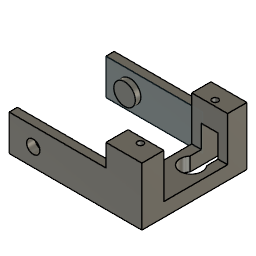
leg connector sprint 5 (Autodesk Fusion 360 design; units mm, degrees)
Autodesk Fusion 360 part; units mm, degrees
sketch "Sketch1" plane through (0, 0, 0) normal (0, 0, 1) x (1, 0, 0)
  line L0 (6.5, -11.5) -> (-6.5, -11.5)
  line L1 (-6.5, -11.5) -> (-6.5, 11.5)
  line L2 (-6.5, 11.5) -> (6.5, 11.5)
  line L3 (6.5, 11.5) -> (6.5, -11.5)
  line L4 (6.5, -11.5) -> (-6.5, 11.5) construction
  line L5 (-6.5, -11.5) -> (6.5, 11.5) construction
  line L6 (6.5, -11.5) -> (-6.5, -11.5)
  line L7 (-6.5, -11.5) -> (-6.5, -17.5)
  line L8 (-6.5, -17.5) -> (6.5, -17.5)
  line L9 (6.5, -17.5) -> (6.5, -11.5)
  line L10 (6.5, 11.5) -> (-6.5, 11.5)
  line L11 (-6.5, 11.5) -> (-6.5, 17.5)
  line L12 (-6.5, 17.5) -> (6.5, 17.5)
  line L13 (6.5, 17.5) -> (6.5, 11.5)
  dimension "d1" = 13
  dimension "d2" = 23
  dimension "d3" = 6
  dimension "d4" = 6
  constraint horizontal L0
  constraint perpendicular L0 L1
  constraint parallel L0 L2
  constraint parallel L1 L3
  constraint coincident L4 origin
  constraint coincident L5 origin
  constraint horizontal L6
  constraint vertical L7
  constraint horizontal L8
  constraint vertical L9
  constraint horizontal L10
  constraint vertical L11
  constraint horizontal L12
  constraint vertical L13
  measures "d1" distance of L1.end L2.end
  measures "d2" distance of L0.end L1.end
  measures "d3" distance of L0.start L8.end
  measures "d4" distance of L2.end L12.end
extrude "Extrude1" add sketch "Sketch1" along normal blind 21 contours L0 L6 L7 L8 L9 | L2 L10 L11 L12 L13 makes body 1 at (-2.1667, -17.5, 7) makes body 2 at (-2.1667, 17.5, 7)
extrude "Extrude2" add sketch "Sketch1" along normal blind 5 contours L0 L1 L2 L3 L6 L10 bodies 1 2
sketch "Sketch2" plane through (0, 0, 5) normal (0, 0, 1) x (-1, 0, 0)
  line L0 (-6.5, 11.5) -> (-6.5, -11.5)
  line L1 (-6.5, -11.5) -> (6.5, -11.5)
  line L2 (6.5, -11.5) -> (6.5, 11.5)
  line L3 (6.5, 11.5) -> (-6.5, 11.5)
  circle A0 centre (0, -5.75) radius 4
  dimension "d9" = 8
  measures "d9" diameter of A0
extrude "Extrude3" cut sketch "Sketch2" against normal blind 6.5 contours A0 bodies 1
sketch "Sketch3" plane through (-6.5, 0, 0) normal (-1, 0, 0) x (0, -1, 0)
  line L0 (-17.5, 0) -> (17.5, 0)
  line L1 (17.5, 0) -> (17.5, 21)
  line L2 (17.5, 21) -> (11.5, 21)
  line L3 (11.5, 21) -> (11.5, 5)
  line L4 (11.5, 5) -> (-11.5, 5)
  line L5 (-11.5, 5) -> (-11.5, 21)
  line L6 (-11.5, 21) -> (-17.5, 21)
  line L7 (-17.5, 21) -> (-17.5, 0)
  line L8 (-17.5, 0) -> (-14.5, 0)
  line L9 (-14.5, 0) -> (-14.5, 13)
  line L10 (-14.5, 13) -> (-17.5, 13)
  line L11 (-17.5, 13) -> (-17.5, 0)
  line L12 (17.5, 0) -> (14.5, 0)
  line L13 (14.5, 0) -> (14.5, 13)
  line L14 (14.5, 13) -> (17.5, 13)
  line L15 (17.5, 13) -> (17.5, 0)
  dimension "d12" = 3
  constraint horizontal L8
  constraint vertical L9
  constraint horizontal L10
  constraint vertical L11
  constraint coincident L0.start L7.end
  constraint horizontal L12
  constraint vertical L13
  constraint horizontal L14
  constraint vertical L15
  constraint coincident L0.end L1.start
  measures "d12" distance of L0.end L12.end
extrude "Extrude4" add sketch "Sketch3" along normal blind 25 contours L0 L7 L8 L9 L10 L11 | L0 L1 L12 L13 L14 L15 bodies 1
chamfer "Chamfer1" distance 2 angle 45 2 edges at (-6.5, 17.5, 17) (-6.5, -17.5, 17) on bodies 1
sketch "Sketch4" plane through (0, -14.5, 0) normal (0, 1, 0) x (-1, 0, 0)
  line L0 (6.5, 13) -> (6.5, 0)
  line L1 (6.5, 0) -> (31.5, 0)
  line L2 (31.5, 0) -> (31.5, 13)
  line L3 (31.5, 13) -> (6.5, 13)
  circle A0 centre (25.25, 6.5) radius 4
  dimension "d16" = 8
  measures "d16" diameter of A0
extrude "Extrude5" add sketch "Sketch4" along normal blind 2 contours A0 bodies 1
sketch "Sketch5" plane through (0, 17.5, 0) normal (0, 1, 0) x (-1, 0, 0)
  line L0 (4.5, 13) -> (4.5, 21)
  line L1 (4.5, 21) -> (-6.5, 21)
  line L2 (-6.5, 21) -> (-6.5, 0)
  line L3 (-6.5, 0) -> (31.5, 0)
  line L4 (31.5, 0) -> (31.5, 13)
  line L5 (31.5, 13) -> (4.5, 13)
  line L6 (-3, -10) -> (3, -10)
  line L7 (3, -10) -> (3, 10)
  line L8 (3, 10) -> (-3, 10)
  line L9 (-3, 10) -> (-3, -10)
  line L10 (-3, -10) -> (3, 10) construction
  line L11 (3, -10) -> (-3, 10) construction
  constraint horizontal L6
  constraint perpendicular L6 L7
  constraint parallel L6 L8
  constraint parallel L7 L9
  constraint coincident L10 origin
  constraint coincident L11 origin
extrude "Extrude6" cut sketch "Sketch5" against normal blind 6 contours L3 L7 L8 L9 bodies 1
extrude "Extrude7" add 2 faces at (-31.5, 16.5, 8.6667) (-31.5, -15.5, 8.6667) along direction (-1, 0, 0) blind 10 on bodies 1 bodies 1
extrude "Extrude8" cut 1 faces at (-26.4956, -12.5, 5.7272) along direction (0, -1, 0) blind 2 on bodies 1 bodies 1
extrude "Extrude9" add 1 faces at (-13.1667, -17.5, 4.3333) along direction (0, -1, 0) blind 5 on bodies 1 bodies 1
extrude "Extrude10" cut 1 faces at (-18.1667, -14.5, 4.3333) along direction (0, -1, 0) blind 2 on bodies 1 bodies 1
extrude "Extrude11" cut 1 faces at (-13.1667, -22.5, 4.3333) along direction (0, 1, 0) blind 3 on bodies 1 bodies 1
sketch "Sketch6" plane through (0, -16.5, 0) normal (0, 1, 0) x (-1, 0, 0)
  line L0 (6.5, 13) -> (6.5, 0)
  line L1 (6.5, 0) -> (41.5, 0)
  line L2 (41.5, 0) -> (41.5, 13)
  line L3 (41.5, 13) -> (6.5, 13)
  line L4 (24, 13) -> (24, 0)
  circle A0 centre (32.75, 6.5) radius 4
  dimension "d31" = 8
  constraint midpoint L3 L4.start
  constraint midpoint L1 L4.end
  measures "d31" diameter of A0
extrude "Extrude12" add sketch "Sketch6" along normal blind 2 contours A0 bodies 1
sketch "Sketch7" plane through (0, 0, 13) normal (0, 0, 1) x (-1, 0, 0)
  line L0 (41.5, 19.5) -> (4.5, 19.5)
  line L1 (4.5, 19.5) -> (4.5, 17.5)
  line L2 (4.5, 17.5) -> (6.5, 15.5)
  line L3 (6.5, 15.5) -> (6.5, 16.5)
  line L4 (6.5, 16.5) -> (41.5, 16.5)
  line L5 (41.5, 16.5) -> (41.5, 19.5)
  line L6 (6.5, 19.5) -> (6.5, 15.5)
  line L7 (6.5, 19.5) -> (4.5, 19.5)
  constraint coincident L0 L6.start
  constraint coincident L2.end L3.start
  constraint coincident L0.end L1.start
extrude "Extrude13" add 1 faces at (-4.5, -18.1667, 15.6667) along direction (-1, 0, 0) blind 2 on bodies 1 bodies 1
extrude "Extrude14" add 1 faces at (-5.8333, -17.5, 15.6667) along direction (0, 1, 0) blind 2 on bodies 1 bodies 1
chamfer "Chamfer2" distance 2 angle 45 1 edges at (-6.5, -19.5, 17) on bodies 1
extrude "Extrude15" cut 1 faces at (-18.1667, 14.5, 4.3333) along direction (0, 1, 0) blind 1 on bodies 1 bodies 1
extrude "Extrude16" add 1 faces at (-16.3333, 17.5, 4.3333) along direction (0, 1, 0) blind 1 on bodies 1 bodies 1
sketch "Sketch8" plane through (0, 15.5, 0) normal (0, -1, 0) x (1, 0, 0)
  line L0 (-6.5, 0) -> (-6.5, 13)
  line L1 (-6.5, 13) -> (-41.5, 13)
  line L2 (-41.5, 13) -> (-41.5, 0)
  line L3 (-41.5, 0) -> (-6.5, 0)
extrude "Extrude17" cut 1 faces at (-31.963, -14.5, 4.8658) along direction (0, 1, 0) blind 38 on bodies 1 bodies 1
sketch "Sketch9" plane through (0, 18.5, 0) normal (0, 1, 0) x (-1, 0, 0)
  circle A0 centre (32.75, 6.5) radius 4
  line L0 (-3, 0) -> (-3, 10)
  line L1 (-3, 10) -> (3, 10)
  line L2 (3, 10) -> (3, 0)
  line L3 (3, 0) -> (41.5, 0)
  line L4 (41.5, 0) -> (41.5, 13)
  line L5 (41.5, 13) -> (4.5, 13)
  line L6 (4.5, 13) -> (4.5, 21)
  line L7 (4.5, 21) -> (-6.5, 21)
  line L8 (-6.5, 21) -> (-6.5, 0)
  line L9 (-6.5, 0) -> (-3, 0)
  circle A1 centre (32.75, 6.5) radius 1.25
  dimension "d45" = 2.5
  constraint concentric A0 A1
  measures "d45" diameter of A1
extrude "Extrude18" add sketch "Sketch9" against normal blind 3 contours A0 bodies 1
extrude "Extrude19" cut 1 faces at (-1, 16.1667, 10) along direction (0, 0, 1) blind 1 on bodies 1 bodies 1
sketch "Sketch10" plane through (0, 0, 21) normal (0, 0, 1) x (-1, 0, 0)
  line L0 (4.5, -17.5) -> (6.5, -15.5)
  line L1 (6.5, -15.5) -> (6.5, -11.5)
  line L2 (6.5, -11.5) -> (-6.5, -11.5)
  line L3 (-6.5, -11.5) -> (-6.5, -18.5)
  line L4 (-6.5, -18.5) -> (4.5, -18.5)
  line L5 (4.5, -18.5) -> (4.5, -17.5)
  circle A0 centre (0, -13.5) radius 1.1
  dimension "d51" = 2.2
  measures "d51" diameter of A0
extrude "Extrude20" cut sketch "Sketch10" against normal blind 4 contours A0 bodies 1
sketch "Sketch11" plane through (0, 0, 21) normal (0, 0, 1) x (-1, 0, 0)
  line L0 (6.5, 17.5) -> (4.5, 19.5)
  line L1 (4.5, 19.5) -> (-6.5, 19.5)
  line L2 (-6.5, 19.5) -> (-6.5, 11.5)
  line L3 (-6.5, 11.5) -> (6.5, 11.5)
  line L4 (6.5, 11.5) -> (6.5, 17.5)
  circle A0 centre (0, 13.5) radius 1.1
  dimension "d55" = 2.2
  measures "d55" diameter of A0
extrude "Extrude21" cut sketch "Sketch11" against normal blind 4 contours A0 bodies 1
sketch "Sketch12" plane through (0, 18.5, 0) normal (0, 1, 0) x (-1, 0, 0)
  line L0 (-3, 0) -> (-3, 11)
  line L1 (-3, 11) -> (3, 11)
  line L2 (3, 11) -> (3, 0)
  line L3 (3, 0) -> (41.5, 0)
  line L4 (41.5, 0) -> (41.5, 13)
  line L5 (41.5, 13) -> (4.5, 13)
  line L6 (4.5, 13) -> (4.5, 21)
  line L7 (4.5, 21) -> (-6.5, 21)
  line L8 (-6.5, 21) -> (-6.5, 0)
  line L9 (-6.5, 0) -> (-3, 0)
  circle A0 centre (32.75, 6.5) radius 1.25
  circle A1 centre (32.75, 6.5) radius 2.4
  dimension "d58" = 4.8
  constraint concentric A0 A1
  measures "d58" diameter of A1
extrude "Extrude22" cut sketch "Sketch12" against normal blind 4.5 contours A1 bodies 1
sketch "Sketch13" plane through (0, 0, 0) normal (0, 0, -1) x (1, 0, 0)
  circle A0 centre (0, -5.75) radius 4
  line L0 (-6.5, 16.5) -> (-6.5, -15.5)
  line L1 (-6.5, -15.5) -> (-41.5, -15.5)
  line L2 (-41.5, -15.5) -> (-41.5, -18.5)
  line L3 (-41.5, -18.5) -> (-3, -18.5)
  line L4 (-3, -18.5) -> (-3, -11.5)
  line L5 (-3, -11.5) -> (3, -11.5)
  line L6 (3, -11.5) -> (3, -18.5)
  line L7 (3, -18.5) -> (6.5, -18.5)
  line L8 (6.5, -18.5) -> (6.5, 19.5)
  line L9 (6.5, 19.5) -> (-41.5, 19.5)
  line L10 (-41.5, 19.5) -> (-41.5, 16.5)
  line L11 (-41.5, 16.5) -> (-6.5, 16.5)
  line L12 (6.5, -11.5) -> (-6.5, -11.5)
  line L13 (-6.5, -11.5) -> (-6.5, 1)
  line L14 (6.5, 1) -> (-6.5, 1)
  line L15 (6.5, 1) -> (6.5, -11.5)
  constraint coincident L8 L12.start
  constraint coincident L0 L12.end
  constraint perpendicular L0 L12
  constraint coincident L0 L13.end
  constraint coincident L8 L14.start
  constraint perpendicular L13 L14
extrude "Extrude23" add sketch "Sketch13" against normal blind 5 contours A0 bodies 1
sketch "Sketch14" plane through (0, 0, 0) normal (0, 0, -1) x (1, 0, 0)
  line L0 (-6.5, 16.5) -> (-6.5, -15.5)
  line L1 (-6.5, -15.5) -> (-41.5, -15.5)
  line L2 (-41.5, -15.5) -> (-41.5, -18.5)
  line L3 (-41.5, -18.5) -> (-3, -18.5)
  line L4 (-3, -18.5) -> (-3, -11.5)
  line L5 (-3, -11.5) -> (3, -11.5)
  line L6 (3, -11.5) -> (3, -18.5)
  line L7 (3, -18.5) -> (6.5, -18.5)
  line L8 (6.5, -18.5) -> (6.5, 19.5)
  line L9 (6.5, 19.5) -> (-41.5, 19.5)
  line L10 (-41.5, 19.5) -> (-41.5, 16.5)
  line L11 (-41.5, 16.5) -> (-6.5, 16.5)
  circle A0 centre (0, -4.8) radius 4
  dimension "d67" = 8
  measures "d67" diameter of A0
extrude "Extrude24" cut sketch "Sketch14" against normal blind 5 contours A0 bodies 1
sketch "Sketch15" plane through (0, 18.5, 0) normal (0, 1, 0) x (-1, 0, 0)
  circle A0 centre (32.75, 6.5) radius 2.4
  line L0 (-3, 0) -> (-3, 11)
  line L1 (-3, 11) -> (3, 11)
  line L2 (3, 11) -> (3, 0)
  line L3 (3, 0) -> (41.5, 0)
  line L4 (41.5, 0) -> (41.5, 13)
  line L5 (41.5, 13) -> (4.5, 13)
  line L6 (4.5, 13) -> (4.5, 21)
  line L7 (4.5, 21) -> (-6.5, 21)
  line L8 (-6.5, 21) -> (-6.5, 0)
  line L9 (-6.5, 0) -> (-3, 0)
  circle A1 centre (32.75, 6.5) radius 2.4
  constraint concentric A0 A1
extrude "Extrude25" cut sketch "Sketch15" against normal blind 49 contours A0 A1 bodies 1
extrude "Extrude26" cut 1 faces at (-36.1928, -14.5, 6.182) along direction (0, -1, 0) blind 2 on bodies 1 bodies 1
sketch "Sketch16" plane through (0, 15.5, 0) normal (0, -1, 0) x (1, 0, 0)
sketch "Sketch17" plane through (0, 15.5, 0) normal (0, -1, 0) x (1, 0, 0)
sketch "Sketch18" plane through (0, 18.5, 0) normal (0, 1, 0) x (-1, 0, 0)
  circle A0 centre (32.75, 6.5) radius 2.4
  line L0 (-3, 0) -> (-3, 11)
  line L1 (-3, 11) -> (3, 11)
  line L2 (3, 11) -> (3, 0)
  line L3 (3, 0) -> (41.5, 0)
  line L4 (41.5, 0) -> (41.5, 13)
  line L5 (41.5, 13) -> (4.5, 13)
  line L6 (4.5, 13) -> (4.5, 21)
  line L7 (4.5, 21) -> (-6.5, 21)
  line L8 (-6.5, 21) -> (-6.5, 0)
  line L9 (-6.5, 0) -> (-3, 0)
  circle A1 centre (32.75, 6.5) radius 4
  dimension "d74" = 8
  constraint concentric A0 A1
  measures "d74" diameter of A1
extrude "Extrude27" add sketch "Sketch18" against normal blind 5 contours A0 | A1 bodies 1
sketch "Sketch19" plane through (0, 0, 13) normal (0, 0, 1) x (-1, 0, 0)
  line L0 (6.5, 17.5) -> (6.5, 16.5)
  line L1 (6.5, 16.5) -> (41.5, 16.5)
  line L2 (41.5, 16.5) -> (41.5, 19.5)
  line L3 (41.5, 19.5) -> (4.5, 19.5)
  line L4 (4.5, 19.5) -> (6.5, 17.5)
  line L5 (6.5, 17.5) -> (6.5, 19.5)
  line L6 (6.5, 19.5) -> (4.5, 19.5)
  constraint coincident L0.start L4.end
  constraint coincident L3 L5.end
  constraint perpendicular L3 L5
  constraint coincident L3.end L4.start
extrude "Extrude28" add sketch "Sketch19" along normal blind 8 contours L3 L4 L5 L6 bodies 1
sketch "Sketch20" plane through (0, 0, 13) normal (0, 0, 1) x (-1, 0, 0)
  line L0 (41.5, -15.5) -> (6.5, -15.5)
  line L1 (6.5, -15.5) -> (4.5, -17.5)
  line L2 (4.5, -17.5) -> (4.5, -18.5)
  line L3 (4.5, -18.5) -> (41.5, -18.5)
  line L4 (41.5, -18.5) -> (41.5, -15.5)
  line L5 (6.5, -15.5) -> (6.5, -18.5)
  line L6 (4.5, -18.5) -> (6.5, -18.5)
  constraint coincident L0.end L1.start
  constraint coincident L3 L5.end
  constraint perpendicular L3 L5
  constraint coincident L2.end L3.start
extrude "Extrude29" add sketch "Sketch20" along normal blind 8 contours L1 L2 L3 L5 L6 bodies 1
extrude "Extrude30" cut 1 faces at (-1, 16.1667, 11) along direction (0, 0, 1) blind 2.2 on bodies 1 bodies 1
sketch "Sketch21" plane through (0, 13.5, 0) normal (0, -1, 0) x (1, 0, 0)
  circle A0 centre (-32.75, 6.5) radius 4
  circle A1 centre (-32.75, 6.5) radius 3.9
  dimension "d83" = 7.8
  constraint concentric A0 A1
  measures "d83" diameter of A1
extrude "Extrude31" cut sketch "Sketch21" against normal blind 2 bodies 1
sketch "Sketch22" plane through (0, 0, 0) normal (0, 0, -1) x (1, 0, 0)
  circle A0 centre (0, -4.8) radius 4
  line L0 (-6.5, 16.5) -> (-6.5, -15.5)
  line L1 (-6.5, -15.5) -> (-41.5, -15.5)
  line L2 (-41.5, -15.5) -> (-41.5, -18.5)
  line L3 (-41.5, -18.5) -> (-3, -18.5)
  line L4 (-3, -18.5) -> (-3, -11.5)
  line L5 (-3, -11.5) -> (3, -11.5)
  line L6 (3, -11.5) -> (3, -18.5)
  line L7 (3, -18.5) -> (6.5, -18.5)
  line L8 (6.5, -18.5) -> (6.5, 19.5)
  line L9 (6.5, 19.5) -> (-41.5, 19.5)
  line L10 (-41.5, 19.5) -> (-41.5, 16.5)
  line L11 (-41.5, 16.5) -> (-6.5, 16.5)
  line L12 (3, -11.5) -> (3, -7.4458)
  line L13 (-3, -11.5) -> (-3, -7.4458)
  line L14 (3, -11.5) -> (3, -7.4425)
  line L15 (3, -7.4425) -> (3, -11.5)
  circle A1 centre (0, -4.8) radius 4
  constraint coincident L5.end L6.start
  constraint coincident A0 L12.end
  constraint perpendicular L5 L12
  constraint coincident L4.end L5.start
  constraint coincident A0 L13.end
  constraint perpendicular L5 L13
  constraint vertical L14
  constraint parallel L14 L15
  constraint concentric A0 A1
extrude "Extrude32" cut sketch "Sketch22" against normal blind 5 contours A0 L5 L12 L13 L14 L15 A1 bodies 1
